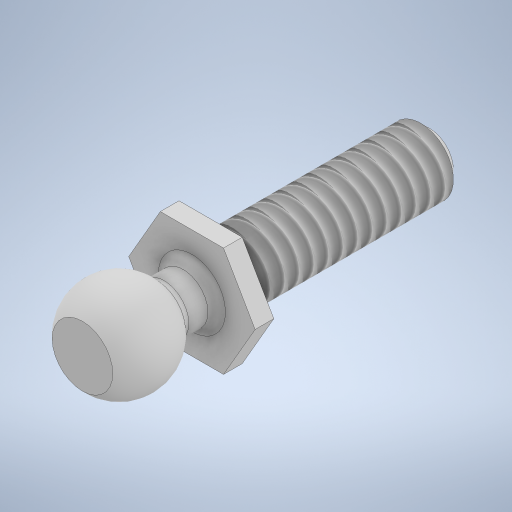
# Autodesk Inventor part: Ball Stud
Saved by Autodesk Inventor 2024 (Build 280153000, 153)
## iProperties
Created: 2023-07-07
Part Number: Ball Stud
Material: Generic
Document SubType Name: Modeling
Designer: birud
Density: 1 g/cm^3
Appearance: Default
Author: birud
Autodesk Inventor part; units mm, degrees
ref_plane "YZ Plane" through (0, 0, 0) normal (1, 0, 0) x (0, 1, 0)
ref_plane "XZ Plane" through (0, 0, 0) normal (0, 1, 0) x (-1, 0, 0)
ref_plane "XY Plane" through (0, 0, 0) normal (0, 0, 1) x (1, 0, 0)
sketch "Sketch1" plane through (0, 0, 0) normal (0, 0, 1) x (1, 0, 0)
  circle A0 centre (0, 0) radius 2.3813 construction
  line L0 (1.3748, 2.3813) -> (2.7496, 0)
  line L1 (2.7496, 0) -> (1.3748, -2.3812)
  line L2 (1.3748, -2.3812) -> (-1.3748, -2.3813)
  line L3 (-1.3748, -2.3813) -> (-2.7496, 0)
  line L4 (-2.7496, 0) -> (-1.3748, 2.3812)
  line L5 (-1.3748, 2.3812) -> (1.3748, 2.3813)
  point P0 (0, 2.3813)
  dimension "d0" = 4.7625
  constraints: 12 end point, 2 coincident, 1 horizontal, 1 midpoint, 1 vertical alignment, 15 other
extrude "Extrusion1" add sketch "Sketch1" along normal blind 0.8128
sketch "Sketch2" plane through (0, 0, 0.8128) normal (0, 0, 1) x (1, 0, 0)
  circle A0 centre (0, 0) radius 1.0795
  dimension "d3" = 2.159
  constraints: 1 centre point, 1 coincident
  measures "d3" diameter of A0
extrude "Extrusion2" add sketch "Sketch2" along normal blind 3.175
sketch "Sketch3" plane through (0, 0, 3.9878) normal (0, 0, 1) x (1, 0, 0)
  circle A0 centre (0, 0) radius 1.0795 projected
  circle A1 centre (0, 0) radius 2.0638
  line L0 (0, 2.0638) -> (0, -2.0638)
  dimension "d6" = 4.1275
  constraints: 2 end point, 2 point on circle, 1 centre point, 1 coincident, 1 midpoint
  measures "d6" diameter of A1
revolve "Revolution1" add sketch "Sketch3" angle 360 about axis through (0, 2.0638, 3.9878) along (0, -1, 0) picked at (-0.2386, -0.2693) picked at (-0.2507, -1.7053) contours L0 A0 | A0 L0 A1
fillet "Fillet1" radius 0.381 2 edges at (-1.0795, 0, 0.8128) (-1.0795, 0, 2.2289)
ref_plane "Work Plane1" through (0, 0, 5.5753) normal (0, 0, 1) x (1, 0, 0)
split "Split1" plane through (0, 0, 5.5753) removes the side toward (0, 0, 1)
sketch "Sketch4" plane through (0, 0, 0) normal (0, 0, -1) x (-1, 0, 0)
  circle A0 centre (0, 0) radius 1.0795 projected
  circle A1 centre (0, 0) radius 1.4224
  dimension "d10" = 2.8448
  constraints: 1 centre point, 1 coincident
  measures "d10" diameter of A1
extrude "Extrusion3" add sketch "Sketch4" along normal blind 9.525 contours A0 | A1
chamfer "Chamfer1" distance 0.381 angle 45 1 edges at (1.4224, 0, -9.525)
thread "Thread1" size "4-40 UNC" class "2A" standard "ANSI Unified Screw Threads" length 26
body "Solid1"
